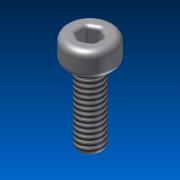
# Autodesk Inventor part: Cap(M2-6)
Saved by Autodesk Inventor 2013 (Build 170138000, 138)
## iProperties
Created: 2014-02-07
Material: 一般
Document SubType Name: Modeling
Designer: andou
Density: 1 g/cm^3
Mass: 0.0373174 g
Surface Area: 0.842779 cm^2
Volume: 0.0373174 cm^3
Author: andou
Title: Cap(M2-6)
Autodesk Inventor part; units mm, degrees
ref_plane "YZ Plane" through (0, 0, 0) normal (1, 0, 0) x (0, 1, 0)
ref_plane "XZ Plane" through (0, 0, 0) normal (0, 1, 0) x (-1, 0, 0)
ref_plane "XY Plane" through (0, 0, 0) normal (0, 0, 1) x (1, 0, 0)
sketch "スケッチ1" plane through (0, 0, 0) normal (0, 0, 1) x (1, 0, 0)
  circle A0 centre (0, 0) radius 1.9
  dimension "d0" = 3.8
  constraints: 1 centre point, 1 coincident
  measures "d0" diameter of A0
extrude "押し出し1" add sketch "スケッチ1" along normal blind 2
sketch "スケッチ2" plane through (0, 0, 0) normal (0, 0, -1) x (-1, 0, 0)
  circle A0 centre (0, 0) radius 1.9 projected
  circle A1 centre (0, 0) radius 1
  dimension "d3" = 2
  constraints: 1 centre point, 1 coincident
  measures "d3" diameter of A1
extrude "押し出し2" add sketch "スケッチ2" along normal blind 6 contours A1
sketch "スケッチ3" plane through (0, 0, 2) normal (0, 0, 1) x (1, 0, 0)
  circle A0 centre (0, 0) radius 1.9 projected
  line L0 (0, 0.866) -> (0.75, 0.433)
  line L1 (0.75, 0.433) -> (0.75, -0.433)
  line L2 (0.75, -0.433) -> (0, -0.866)
  line L3 (0, -0.866) -> (-0.75, -0.433)
  line L4 (-0.75, -0.433) -> (-0.75, 0.433)
  line L5 (-0.75, 0.433) -> (0, 0.866)
  dimension "d6" = 0.75
  constraints: 12 end point, 1 coincident, 13 other
  measures "d6" distance from line of point (0, 0) L0
extrude "押し出し3" cut sketch "スケッチ3" against normal blind 1.5 contours L0 L1 L2 L3 L4 L5
fillet "フィレット1" radius 0.5 2 edges at (-1.9, 0, 2) (-1.9, 0, 0)
fillet "フィレット2" radius 0.3 19 edges at (-0.375, 0.6495, 2) (-0.75, 0, 2) (-0.375, -0.6495, 2) (0.375, -0.6495, 2) (0.75, 0, 2) (0.375, 0.6495, 2) (-0.375, 0.6495, 0.5) (0.375, 0.6495, 0.5) (0, 0.866, 1.25) (-0.75, 0.433, 1.25) (-0.375, -0.6495, 0.5) (-0.75, -0.433, 1.25) (-0.75, 0, 0.5) (0.75, 0, 0.5) (0.75, 0.433, 1.25) (0.75, -0.433, 1.25) (0.375, -0.6495, 0.5) (0, -0.866, 1.25) (1, 0, -6)
thread "ねじ3" size "M2x0.4" class "6g" standard "ANSI Metric M Profile" full length
